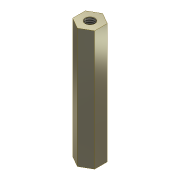
# Autodesk Inventor part: 黄銅スペーサー（六角）_ASB-330E
Saved by Autodesk Inventor 2016 (Build 200138000, 138)
## iProperties
Created: 2016-11-01
Part Number: 黄銅スペーサー（六角）_ASB-330E
Material: 真鍮、ソフト イエロー
Document SubType Name: Modeling
Designer: NN
Density: 8.47 g/cm^3
Appearance: ニッケル
Mass: 5.92896 g
Surface Area: 7.61517 cm^2
Volume: 0.699996 cm^3
Author: NN
Autodesk Inventor part; units mm, degrees
ref_plane "YZ Plane" through (0, 0, 0) normal (1, 0, 0) x (0, 1, 0)
ref_plane "XZ Plane" through (0, 0, 0) normal (0, 1, 0) x (-1, 0, 0)
ref_plane "XY Plane" through (0, 0, 0) normal (0, 0, 1) x (1, 0, 0)
sketch "スケッチ1" plane through (0, 0, 0) normal (0, 0, 1) x (1, 0, 0)
  line L0 (0, 3.1754) -> (2.75, 1.5877)
  line L1 (2.75, 1.5877) -> (2.75, -1.5877)
  line L2 (2.75, -1.5877) -> (0, -3.1754)
  line L3 (0, -3.1754) -> (-2.75, -1.5877)
  line L4 (-2.75, -1.5877) -> (-2.75, 1.5877)
  line L5 (-2.75, 1.5877) -> (0, 3.1754)
  point P0 (0, 0)
  point P1 (0, 0)
  dimension "d0" = 5.5
  constraints: 12 end point, 1 coincident, 1 vertical, 13 other
  measures "d0" distance between parallel lines of L1 L4
extrude "押し出し1" add sketch "スケッチ1" along normal blind 30
sketch "スケッチ2" plane through (0, 0, 30) normal (0, 0, 1) x (1, 0, 0)
  line L0 (2.75, 1.5877) -> (0, 3.1754) projected
  line L1 (0, 3.1754) -> (-2.75, 1.5877) projected
  line L2 (-2.75, 1.5877) -> (-2.75, -1.5877) projected
  line L3 (-2.75, -1.5877) -> (0, -3.1754) projected
  line L4 (0, -3.1754) -> (2.75, -1.5877) projected
  line L5 (2.75, -1.5877) -> (2.75, 1.5877) projected
  point P0 (0, 0)
hole "穴1" at (0, 0, 30) direction (0, 0, -1) diameter 2.459 depth 8.8 tip angle 118 thread size "M3x0.5" class "6H" standard "ISO Metric profile"
sketch "スケッチ3" plane through (0, 0, 0) normal (0, 0, -1) x (-1, 0, 0)
  line L0 (0, 3.1754) -> (-2.75, 1.5877) projected
  line L1 (-2.75, 1.5877) -> (-2.75, -1.5877) projected
  line L2 (-2.75, -1.5877) -> (0, -3.1754) projected
  line L3 (0, -3.1754) -> (2.75, -1.5877) projected
  line L4 (2.75, -1.5877) -> (2.75, 1.5877) projected
  line L5 (2.75, 1.5877) -> (0, 3.1754) projected
  point P0 (0, 0)
hole "穴2" at (0, 0, 0) direction (0, 0, 1) diameter 2.459 depth 8.8 tip angle 118 thread size "M3x0.5" class "6H" standard "ISO Metric profile"
